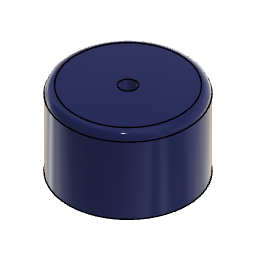
base v4 (Autodesk Fusion 360 design; units mm, degrees)
Autodesk Fusion 360 part; units mm, degrees
sketch "Sketch1" plane through (0, 0, 0) normal (0, 0, 1) x (1, 0, 0)
  circle A0 centre (0, 0) radius 200
  dimension "d1" = 400
  constraint coincident A0.centre origin
  measures "d1" diameter of A0
extrude "Extrude1" add sketch "Sketch1" along normal blind 250
sketch "Sketch2" plane through (0, 0, 250) normal (0, 0, 1) x (-1, 0, 0)
  circle A0 centre (0, 0) radius 200
  circle A1 centre (0, 0) radius 25
  dimension "d4" = 50
  constraint concentric A0 A1
  measures "d4" diameter of A1
extrude "Extrude2" cut sketch "Sketch2" against normal blind 75 contours A1
fillet "Fillet1" radius 25 1 edges at (-186.4655, -72.3231, 250)
scale "Scale1" factor 2.5 about (0, 0, 0) bodies 1
